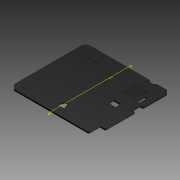
# Autodesk Inventor part: D-054
Saved by Autodesk Inventor 2015 (Build 190159000, 159)
## iProperties
Company: MARCHA TECHNOLOGY
Created: 2013-10-02
Part Number: D-054
Document SubType Name: Modeling
Designer: O.Martin
Density: 1.06 g/cm^3
Material: ABS Plastic
Mass: 736.814 g
Surface Area: 2028.63 cm^2
Volume: 695.108 cm^3
Project: WITBOXprinter_K01
Description: TAPA TRASERA
Stock Number: 28655
Appearance: Black Cast
Author: O.Martin
Autodesk Inventor part; units mm, degrees
ref_plane "XZ Plane" through (0, 0, 0) normal (0, 1, 0) x (-1, 0, 0)
ref_plane "XY Plane" through (0, 0, 0) normal (0, 0, 1) x (1, 0, 0)
sketch "Boceto1" plane through (0, 0, 0) normal (0, 0, 1) x (1, 0, 0)
  line L0 (-240, 218.25) -> (240, 218.25)
  line L1 (240, 218.25) -> (240, -218.25)
  line L2 (240, -218.25) -> (-240, -218.25)
  line L3 (-240, -218.25) -> (-240, 218.25)
  line L4 (-240, 193.25) -> (-215, 218.25)
  line L5 (240, 193.25) -> (215, 218.25)
  line L6 (-240, -193.25) -> (-215, -218.25)
  line L7 (240, -193.25) -> (215, -218.25)
  point P0 (0, 218.25)
  point P1 (240, 0)
  point P2 (0, -218.25)
  dimension "d0" = 480
  dimension "d1" = 436.5
  dimension "d9" = 25
  constraints: 16 end point, 8 point on line, 6 perpendicular, 3 midpoint, 3 parallel, 1 horizontal
  measures "d0" distance of L0.start L0.end
  measures "d1" distance of L0.end L1.end
  measures "d9" horizontal distance of L4.start L4.end
extrude "Extrusión1" add sketch "Boceto1" along normal blind 8 contours L0 L5 L1 L7 L2 L6 L3 L4
sketch "Boceto11" plane through (0, 0, 8) normal (0, 0, 1) x (1, 0, 0)
  line L0 (-198.5, 182.25) -> (198.5, 182.25) construction
  line L1 (198.5, 182.25) -> (198.5, -182.25) construction
  line L2 (198.5, -182.25) -> (-198.5, -182.25) construction
  line L3 (-198.5, -182.25) -> (-198.5, 182.25) construction
  line L4 (240, -193.25) -> (240, 193.25) construction
  line L5 (-215, -218.25) -> (215, -218.25) construction
  line L6 (-215, 218.25) -> (215, 218.25)
  point P0 (198.5, 0)
  point P1 (0, 182.25)
  point P2 (-198.5, 0)
  point P3 (198.5, 0)
  point P4 (0, 182.25)
  point P5 (0, -182.25)
  point P6 (0, 218.25)
  dimension "d67" = 36
  dimension "d95" = 364.5
  dimension "d106" = 397
  constraints: 14 end point, 6 coincident, 5 midpoint, 2 parallel, 1 horizontal, 1 perpendicular, 1 vertical alignment
  measures "d67" distance between parallel lines of L5 L2
  measures "d95" distance of L0.end L1.end
  measures "d106" distance of L1.end L2.end
hole "Agujero1" at (-198.5, 182.25, 8) at (198.5, 182.25, 8) at (198.5, -182.25, 8) at (-198.5, -182.25, 8) at (0, 182.25, 8) direction (0, 0, -1) diameter 6.5 end through all
sketch "Boceto16" plane through (0, 0, 0) normal (0, 0, -1) x (-1, 0, 0)
  line L0 (215, 218.25) -> (240, 193.25) projected
  line L1 (-215, 218.25) -> (215, 218.25) projected
  line L2 (-240, 193.25) -> (-215, 218.25) projected
  line L3 (215, -218.25) -> (-215, -218.25) projected
  line L4 (-222, 211.25) -> (222, 211.25)
  dimension "d96" = 7
  constraints: 2 end point, 2 point on line, 1 parallel
  measures "d96" distance between parallel lines of L1 L4
extrude "Extrusión11" cut sketch "Boceto16" against normal through all
sketch "Boceto17" plane through (0, 0, 0) normal (0, 0, -1) x (-1, 0, 0)
  line L0 (-160, 11.75) -> (-120, 11.75)
  line L1 (-120, 11.75) -> (-120, -18.25)
  line L2 (-120, -18.25) -> (-160, -18.25)
  line L3 (-160, -18.25) -> (-160, 11.75)
  circle A0 centre (-198.5, 182.25) radius 3.25 projected
  line L4 (-160, -3.25) -> (-120, -3.25) construction
  point P0 (-140, 11.75)
  dimension "d117" = 40
  dimension "d118" = 30
  dimension "d120" = 170.5
  constraints: 10 end point, 3 midpoint, 2 parallel, 1 horizontal, 1 perpendicular
  measures "d117" distance of L0.start L0.end
  measures "d118" distance of L2.end L0.start
  measures "d120" distance from line of A0.centre L0
sketch "Boceto18" plane through (0, 0, 0) normal (0, 0, -1) x (-1, 0, 0)
  line L0 (-240, -193.25) -> (-240, 193.25) projected
  line L1 (-215, -218.25) -> (-240, -193.25) projected
  line L2 (215, -218.25) -> (-215, -218.25) projected
  line L3 (240, 193.25) -> (240, -193.25) projected
  line L4 (-208.5, -218.25) -> (-208.5, -155.25)
  line L5 (-208.5, -155.25) -> (-240, -155.25)
  dimension "d108" = 31.5
  dimension "d109" = 63
  constraints: 4 end point, 2 point on line, 1 parallel, 1 perpendicular
  measures "d108" distance between parallel lines of L4 L0
  measures "d109" distance between parallel lines of L5 L2
extrude "Extrusión13" cut sketch "Boceto18" against normal through all
fillet "Empalme5" radius 2 1 edges at (208.5, -155.25, 4)
chamfer "Chaflán5" distance 5 angle 45 2 edges at (240, -155.25, 4) (208.5, -218.25, 4)
sketch "Boceto19" plane through (0, 0, 8) normal (0, 0, 1) x (1, 0, 0)
  line L0 (222, 211.25) -> (-222, 211.25) projected
  line L1 (203.5, -218.25) -> (-215, -218.25) projected
  line L2 (75, 114.25) -> (-75, 114.25) construction
  line L3 (-75, 114.25) -> (-75, -185.75) construction
  line L4 (-75, -185.75) -> (75, -185.75) construction
  line L5 (75, -185.75) -> (75, 114.25) construction
  line L6 (12.5, -164) -> (-12.5, -164) construction
  line L7 (-12.5, -164) -> (-12.5, -141.5) construction
  line L8 (-12.5, -141.5) -> (12.5, -141.5) construction
  line L9 (12.5, -141.5) -> (12.5, -164) construction
  line L10 (122, 11.75) -> (158, 11.75) projected
  circle A0 centre (198.5, 182.25) radius 3.25 projected
  line L11 (198.5, 108.75) -> (198.5, 78.75) construction
  line L12 (120, -16.25) -> (120, 9.75) projected
  line L13 (15, 39.25) -> (33.75, 39.25) construction
  circle A1 centre (198.5, -182.25) radius 3.25 projected
  circle A2 centre (0, 182.25) radius 3.25 projected
  point P0 (0, 211.25)
  point P1 (0, 114.25)
  point P2 (0, -141.5)
  dimension "d122" = 150
  dimension "d123" = 300
  dimension "d124" = 32.5
  dimension "d125" = 22.5
  dimension "d126" = 25
  dimension "d127" = 21.75
  dimension "d145" = 30
  dimension "d146" = 73.5
  dimension "d147" = 18.75
  dimension "d180" = 221.5
  dimension "d181" = 15
  constraints: 20 end point, 10 coincident, 4 parallel, 4 perpendicular, 3 midpoint, 3 vertical alignment, 2 horizontal
  measures "d122" distance of L2.start L2.end
  measures "d123" distance of L2.end L3.end
  measures "d124" distance between parallel lines of L1 L4
  measures "d125" distance of L6.end L7.end
  measures "d126" distance of L7.end L8.end
  measures "d127" distance between parallel lines of L4 L6
  measures "d145" distance of L11.start L11.end
  measures "d146" distance of A0.centre L11.start
  measures "d147" distance of L13.start L13.end
  measures "d180" distance from line of A1.centre L13
  measures "d181" horizontal distance of A2.centre point (15, 39.25)
hole "Agujero2" [suppressed]
pattern_linear "Patrón rectangular1" [suppressed]
hole "Agujero3" [suppressed]
sketch "Boceto20" plane through (0, 0, 8) normal (0, 0, 1) x (1, 0, 0)
  line L0 (240, 193.25) -> (240, -150.25) projected
  circle A0 centre (198.5, 182.25) radius 3.25 projected
  circle A1 centre (0, 182.25) radius 3.25 projected
  line L1 (7.5, 99.55) -> (-7.5, 99.55)
  line L2 (-7.5, 99.55) -> (-7.5, 132.55)
  line L3 (-7.5, 132.55) -> (7.5, 132.55)
  line L4 (7.5, 132.55) -> (7.5, 99.55)
  line L5 (240, 12.5) -> (222, 12.5)
  line L6 (222, 12.5) -> (222, 57.5)
  line L7 (222, 57.5) -> (240, 57.5)
  line L8 (240, 57.5) -> (240, 12.5)
  line L9 (7.5, 116.05) -> (-7.5, 116.05) construction
  point P0 (0, 99.55)
  point P1 (240, 35)
  dimension "d150" = 15
  dimension "d151" = 66.2
  dimension "d152" = 33
  dimension "d153" = 18
  dimension "d154" = 147.25
  dimension "d155" = 45
  constraints: 18 end point, 4 midpoint, 4 parallel, 2 horizontal, 2 perpendicular, 1 point on line, 1 vertical alignment
  measures "d150" distance of L2.end L3.end
  measures "d151" distance from line of L9 A1.centre
  measures "d152" distance of L3.end L1.start
  measures "d153" distance of L5.start L5.end
  measures "d154" vertical distance of A0.centre point (240, 35)
  measures "d155" distance of L5.end L6.end
extrude "Extrusión14" cut sketch "Boceto20" against normal through all contours L0 L5 L6 L7 | L1 L2 L3 L4
fillet "Empalme7" radius 4 8 edges at (222, 57.5, 4) (222, 12.5, 4) (7.5, 132.55, 4) (7.5, 99.55, 4) (-7.5, 99.55, 4) (-7.5, 132.55, 4) (240, 57.5, 4) (240, 12.5, 4)
sketch "Boceto21" plane through (0, 0, 0) normal (0, 0, -1) x (-1, 0, 0)
  line L0 (222, 211.25) -> (-222, 211.25) projected
  circle A0 centre (-198.5, 182.25) radius 3.25 projected
  circle A1 centre (-152.5, 206.25) radius 5
  line L1 (-156.0355, 202.7145) -> (-164.5711, 211.25)
  line L2 (-148.9645, 202.7145) -> (-140.4289, 211.25)
  line L3 (-240, 193.25) -> (-222, 211.25) projected
  line L4 (3.5, 99.55) -> (-3.5, 99.55) projected
  line L5 (-152.5, 201.25) -> (-137.5, 201.25)
  arc A2 (-137.5, 201.25) -> (-133.9645, 202.7145) centre (-137.5, 206.25) ccw
  line L6 (-133.9645, 202.7145) -> (-125.4289, 211.25)
  dimension "d159" = 5
  dimension "d161" = 46
  dimension "d162" = 10
  dimension "d165" = 45
  dimension "d166" = 90
  dimension "d176" = 15
  constraints: 8 end point, 5 point on circle, 5 tangent, 3 point on line, 2 centre point, 2 parallel, 1 horizontal alignment
  measures "d159" distance from line of L0 A1.centre
  measures "d161" horizontal distance of A1.centre A0.centre
  measures "d162" diameter of A1
  measures "d165" angle of L0 L1
  measures "d166" angle of L1 L2
  measures "d176" distance of A1.centre A2.centre
extrude "Extrusión15" cut sketch "Boceto21" against normal through all contours L6 A2 L5 A1 L2 L0 | L2 A1 L0 | A1 L1 L0 | A1
sketch "Boceto23" plane through (0, 0, 0) normal (0, 0, -1) x (-1, 0, 0)
  line L0 (175.75, 69) -> (104.25, 69) projected
  line L1 (0.0587, -128.1975) -> (14.8322, -128.1975)
  line L2 (14.8322, -128.1975) -> (33.9252, -153.0897)
  circle A0 centre (0, -141.5) radius 1.621 construction
  circle A1 centre (-12.5, -164) radius 1.621 construction
  circle A2 centre (12.5, -164) radius 1.621 construction
  circle A3 centre (0, -141.5) radius 7.5
  circle A4 centre (12.5, -164) radius 7.5
  circle A5 centre (-12.5, -164) radius 7.5
  line L3 (-19.0562, -160.3577) -> (-6.5562, -137.8577)
  line L4 (6.5562, -137.8577) -> (19.0562, -160.3577)
  line L5 (-12.5, -171.5) -> (12.5, -171.5)
  line L6 (215, -218.25) -> (-203.5, -218.25) projected
  line L7 (-19.0562, -160.3577) -> (-51.2186, -218.25)
  line L8 (19.0562, -160.3577) -> (51.2186, -218.25)
  dimension "d177" = 15
  constraints: 14 end point, 8 tangent, 6 point on circle, 3 centre point, 3 coincident, 2 collinear, 2 equal radius, 2 point on line, 1 parallel
  measures "d177" diameter of A3
extrude "Extrusión17" cut sketch "Boceto23" against normal through all contours A3 | A3 L4 A4 L5 A5 L3 | A4 | A5
sketch "Boceto24" plane through (0, 0, 0) normal (0, 0, -1) x (-1, 0, 0)
  line L0 (-35, -167.7147) -> (35, -167.7147) construction
  line L1 (35, -167.7147) -> (35, -217.7147) construction
  line L2 (35, -217.7147) -> (-35, -217.7147) construction
  line L3 (-35, -217.7147) -> (-35, -167.7147) construction
  arc A0 (6.5562, -137.8577) -> (-6.5562, -137.8577) centre (0, -141.5) ccw projected
  point P0 (0, -167.7147)
  dimension "d182" = 70
  dimension "d183" = 50
  constraints: 8 end point, 2 parallel, 1 midpoint, 1 perpendicular, 1 vertical alignment
  measures "d182" distance of L0.start L0.end
  measures "d183" distance of L0.end L1.end
extrude "Extrusión18" [suppressed]
sketch "Boceto25" plane through (0, 0, 0) normal (0, 0, -1) x (-1, 0, 0)
  circle A0 centre (-198.5, 182.25) radius 3.25 projected
  line L0 (-206, 116.25) -> (-191, 116.25)
  line L1 (-191, 116.25) -> (-191, 71.25)
  line L2 (-191, 71.25) -> (-206, 71.25)
  line L3 (-206, 71.25) -> (-206, 116.25)
  line L4 (-206, 93.75) -> (-191, 93.75) construction
  point P0 (-198.5, 116.25)
  dimension "d188" = 15
  dimension "d190" = 45
  dimension "d193" = 88.5
  constraints: 10 end point, 3 midpoint, 2 parallel, 1 horizontal, 1 perpendicular, 1 vertical alignment
  measures "d188" distance of L1.end L2.end
  measures "d190" distance of L2.end L0.start
  measures "d193" distance from line of A0.centre L4
extrude "Extrusión19" cut sketch "Boceto25" against normal through all contours L0 L1 L2 L3
fillet "Empalme9" radius 4 4 edges at (206, 116.25, 4) (191, 116.25, 4) (191, 71.25, 4) (206, 71.25, 4)
extrude "Extrusión20" cut sketch "Boceto17" against normal up to next contours L0 L1 L2 L3
sketch "Boceto26" plane through (0, 0, 0) normal (0, 0, -1) x (-1, 0, 0)
  line L0 (-178.25, 138.25) -> (-178.25, 83.25) projected
  arc A0 (-173.25, 138.25) -> (-178.25, 138.25) centre (-175.75, 138.25) ccw projected
  line L1 (-173.25, 138.25) -> (-173.25, 83.25) projected
  arc A1 (-178.25, 83.25) -> (-173.25, 83.25) centre (-175.75, 83.25) ccw projected
  circle A2 centre (-175.75, 75) radius 2.625 projected
  circle A3 centre (-175.75, 146.5) radius 2.625 projected
  line L2 (-169.5, 75) -> (-169.5, 146.5) projected
  arc A4 (-164.5, 146.5) -> (-169.5, 146.5) centre (-167, 146.5) ccw projected
  line L3 (-164.5, 146.5) -> (-164.5, 75) projected
  line L4 (-160.5, 75) -> (-160.5, 146.5) projected
  arc A5 (-155.5, 146.5) -> (-160.5, 146.5) centre (-158, 146.5) ccw projected
  line L5 (-155.5, 146.5) -> (-155.5, 75) projected
  line L6 (-151.5, 75) -> (-151.5, 146.5) projected
  arc A6 (-146.5, 146.5) -> (-151.5, 146.5) centre (-149, 146.5) ccw projected
  line L7 (-146.5, 146.5) -> (-146.5, 75) projected
  line L8 (-142.5, 75) -> (-142.5, 146.5) projected
  arc A7 (-137.5, 146.5) -> (-142.5, 146.5) centre (-140, 146.5) ccw projected
  line L9 (-137.5, 146.5) -> (-137.5, 75) projected
  line L10 (-133.5, 75) -> (-133.5, 146.5) projected
  arc A8 (-128.5, 146.5) -> (-133.5, 146.5) centre (-131, 146.5) ccw projected
  line L11 (-128.5, 146.5) -> (-128.5, 75) projected
  arc A9 (-119.5, 146.5) -> (-124.5, 146.5) centre (-122, 146.5) ccw projected
  line L12 (-124.5, 75) -> (-124.5, 146.5) projected
  line L13 (-119.5, 146.5) -> (-119.5, 75) projected
  line L14 (-115.5, 75) -> (-115.5, 146.5) projected
  arc A10 (-110.5, 146.5) -> (-115.5, 146.5) centre (-113, 146.5) ccw projected
  line L15 (-110.5, 146.5) -> (-110.5, 75) projected
  arc A11 (-101.75, 138.25) -> (-106.75, 138.25) centre (-104.25, 138.25) ccw projected
  line L16 (-106.75, 83.25) -> (-106.75, 138.25) projected
  line L17 (-101.75, 138.25) -> (-101.75, 83.25) projected
  circle A12 centre (-104.25, 146.5) radius 2.625 projected
  arc A13 (-106.75, 83.25) -> (-101.75, 83.25) centre (-104.25, 83.25) ccw projected
  circle A14 centre (-104.25, 75) radius 2.625 projected
  line L18 (178.25, 138.25) -> (178.25, 83.25) projected
  line L19 (169.5, 146.5) -> (169.5, 75) projected
  line L20 (173.25, 83.25) -> (173.25, 138.25) projected
  circle A15 centre (175.75, 146.5) radius 2.625 projected
  arc A16 (178.25, 138.25) -> (173.25, 138.25) centre (175.75, 138.25) ccw projected
  arc A17 (173.25, 83.25) -> (178.25, 83.25) centre (175.75, 83.25) ccw projected
  arc A18 (164.5, 75) -> (169.5, 75) centre (167, 75) ccw projected
  line L21 (160.5, 75) -> (160.5, 146.5) projected
  arc A19 (169.5, 146.5) -> (164.5, 146.5) centre (167, 146.5) ccw projected
  line L22 (164.5, 75) -> (164.5, 146.5) projected
  arc A20 (155.5, 75) -> (160.5, 75) centre (158, 75) ccw projected
  line L23 (155.5, 75) -> (155.5, 146.5) projected
  arc A21 (160.5, 146.5) -> (155.5, 146.5) centre (158, 146.5) ccw projected
  line L24 (-160, -18.25) -> (-160, 11.75) projected
  line L25 (-160, 11.75) -> (-120, 11.75) projected
  line L26 (-120, 11.75) -> (-120, -18.25) projected
  line L27 (-120, -18.25) -> (-160, -18.25) projected
  line L28 (-206, 75.25) -> (-206, 112.25) projected
  arc A22 (-202, 116.25) -> (-206, 112.25) centre (-202, 112.25) ccw projected
  line L29 (-202, 116.25) -> (-195, 116.25) projected
  arc A23 (-191, 112.25) -> (-195, 116.25) centre (-195, 112.25) ccw projected
  line L30 (-191, 112.25) -> (-191, 75.25) projected
  arc A24 (-195, 71.25) -> (-191, 75.25) centre (-195, 75.25) ccw projected
  line L31 (-195, 71.25) -> (-202, 71.25) projected
  arc A25 (-206, 75.25) -> (-202, 71.25) centre (-202, 75.25) ccw projected
  line L32 (-19.0562, -160.3577) -> (-6.5562, -137.8577) projected
  arc A26 (6.5562, -137.8577) -> (-6.5562, -137.8577) centre (0, -141.5) ccw projected
  line L33 (6.5562, -137.8577) -> (19.0562, -160.3577) projected
  arc A27 (12.5, -171.5) -> (19.0562, -160.3577) centre (12.5, -164) ccw projected
  line L34 (12.5, -171.5) -> (-12.5, -171.5) projected
  arc A28 (-19.0562, -160.3577) -> (-12.5, -171.5) centre (-12.5, -164) ccw projected
  line L35 (-7.5, 103.55) -> (-7.5, 128.55) projected
  arc A29 (-3.5, 132.55) -> (-7.5, 128.55) centre (-3.5, 128.55) ccw projected
  line L36 (-3.5, 132.55) -> (3.5, 132.55) projected
  arc A30 (7.5, 128.55) -> (3.5, 132.55) centre (3.5, 128.55) ccw projected
  line L37 (7.5, 128.55) -> (7.5, 103.55) projected
  arc A31 (3.5, 99.55) -> (7.5, 103.55) centre (3.5, 103.55) ccw projected
  line L38 (3.5, 99.55) -> (-3.5, 99.55) projected
  arc A32 (-7.5, 103.55) -> (-3.5, 99.55) centre (-3.5, 103.55) ccw projected
  circle A33 centre (198.5, 182.25) radius 3.25 projected
  circle A34 centre (-198.5, 182.25) radius 3.25 projected
  circle A35 centre (-198.5, -182.25) radius 3.25 projected
  circle A36 centre (198.5, -182.25) radius 3.25 projected
  circle A37 centre (0, 182.25) radius 3.25 projected
  line L39 (-125.4289, 211.25) -> (-133.9645, 202.7145) projected
  arc A38 (-137.5, 201.25) -> (-133.9645, 202.7145) centre (-137.5, 206.25) ccw projected
  line L40 (-137.5, 201.25) -> (-152.5, 201.25) projected
  arc A39 (-156.0355, 202.7145) -> (-152.5, 201.25) centre (-152.5, 206.25) ccw projected
  line L41 (-156.0355, 202.7145) -> (-164.5711, 211.25) projected
  line L42 (-164.5711, 211.25) -> (-222, 211.25) projected
  line L43 (-240, 193.25) -> (-222, 211.25) projected
  line L44 (-240, 61.5) -> (-240, 193.25) projected
  arc A40 (-240, 61.5) -> (-236, 57.5) centre (-236, 61.5) ccw projected
  line L45 (-236, 57.5) -> (-226, 57.5) projected
  arc A41 (-222, 53.5) -> (-226, 57.5) centre (-226, 53.5) ccw projected
  line L46 (-222, 53.5) -> (-222, 16.5) projected
  arc A42 (-226, 12.5) -> (-222, 16.5) centre (-226, 16.5) ccw projected
  line L47 (-226, 12.5) -> (-236, 12.5) projected
  arc A43 (-236, 12.5) -> (-240, 8.5) centre (-236, 8.5) ccw projected
  line L48 (-240, -150.25) -> (-240, 8.5) projected
  line L49 (-235, -155.25) -> (-240, -150.25) projected
  line L50 (-235, -155.25) -> (-210.5, -155.25) projected
  arc A44 (-208.5, -157.25) -> (-210.5, -155.25) centre (-210.5, -157.25) ccw projected
  line L51 (-208.5, -157.25) -> (-208.5, -213.25) projected
  line L52 (-203.5, -218.25) -> (-208.5, -213.25) projected
  line L53 (215, -218.25) -> (-203.5, -218.25) projected
  line L54 (240, -193.25) -> (215, -218.25) projected
  line L55 (240, 193.25) -> (240, -193.25) projected
  line L56 (222, 211.25) -> (240, 193.25) projected
  line L57 (222, 211.25) -> (-125.4289, 211.25) projected
  arc A45 (151.5, 146.5) -> (146.5, 146.5) centre (149, 146.5) ccw projected
  line L58 (151.5, 146.5) -> (151.5, 75) projected
  line L59 (146.5, 75) -> (146.5, 146.5) projected
  arc A46 (146.5, 75) -> (151.5, 75) centre (149, 75) ccw projected
  arc A47 (137.5, 75) -> (142.5, 75) centre (140, 75) ccw projected
  line L60 (142.5, 146.5) -> (142.5, 75) projected
  line L61 (137.5, 75) -> (137.5, 146.5) projected
  arc A48 (142.5, 146.5) -> (137.5, 146.5) centre (140, 146.5) ccw projected
  arc A49 (133.5, 146.5) -> (128.5, 146.5) centre (131, 146.5) ccw projected
  line L62 (133.5, 146.5) -> (133.5, 75) projected
  line L63 (128.5, 75) -> (128.5, 146.5) projected
  arc A50 (128.5, 75) -> (133.5, 75) centre (131, 75) ccw projected
  line L64 (124.5, 146.5) -> (124.5, 75) projected
  line L65 (119.5, 75) -> (119.5, 146.5) projected
  arc A51 (119.5, 75) -> (124.5, 75) centre (122, 75) ccw projected
  line L66 (115.5, 146.5) -> (115.5, 75) projected
  line L67 (110.5, 75) -> (110.5, 146.5) projected
  arc A52 (110.5, 75) -> (115.5, 75) centre (113, 75) ccw projected
  arc A53 (115.5, 146.5) -> (110.5, 146.5) centre (113, 146.5) ccw projected
  arc A54 (124.5, 146.5) -> (119.5, 146.5) centre (122, 146.5) ccw projected
  circle A55 centre (104.25, 146.5) radius 2.625 projected
  arc A56 (106.75, 138.25) -> (101.75, 138.25) centre (104.25, 138.25) ccw projected
  line L68 (101.75, 83.25) -> (101.75, 138.25) projected
  line L69 (106.75, 138.25) -> (106.75, 83.25) projected
  arc A57 (101.75, 83.25) -> (106.75, 83.25) centre (104.25, 83.25) ccw projected
  circle A58 centre (104.25, 75) radius 2.625 projected
  circle A59 centre (175.75, 75) radius 2.625 projected
  arc A60 (-169.5, 75) -> (-164.5, 75) centre (-167, 75) ccw
  arc A61 (-160.5, 75) -> (-155.5, 75) centre (-158, 75) ccw
  arc A62 (-151.5, 75) -> (-146.5, 75) centre (-149, 75) ccw
  arc A63 (-142.5, 75) -> (-137.5, 75) centre (-140, 75) ccw
  arc A64 (-133.5, 75) -> (-128.5, 75) centre (-131, 75) ccw
  arc A65 (-124.5, 75) -> (-119.5, 75) centre (-122, 75) ccw
  arc A66 (-115.5, 75) -> (-110.5, 75) centre (-113, 75) ccw
  constraints: 14 point on circle, 14 tangent, 7 centre point
extrude "Extrusión21" cut sketch "Boceto26" against normal up to next contours A0 L1 A1 L0 | A2 | A3 | L2 A4 L3 A60 | L4 A5 L5 A61 | L6 A6 L7 A62 | L8 A7 L9 A63 | L10 A8 L11 A64 | L13 A65 L12 A9 | L14 A10 L15 A66 | L17 A13 L16 A11 | A12 | A14 | L18 A17 L20 A16 | L19 A18 L22 A19 | A15 | A20 L23 A21 L21 | L58 A46 L59 A45 | L61 A48 L60 A47 | L62 A50 L63 A49 | L64 A51 L65 A54 | L66 A52 L67 A53 | A55 | L69 A57 L68 A56 | A58 | A59
body "Solid1"
